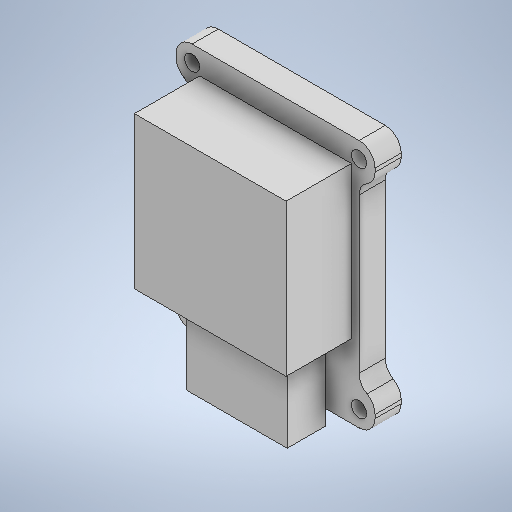
# Autodesk Inventor part: IR_cam
Saved by Autodesk Inventor 2025.3 (Build 293356000, 356)
## iProperties
Created: 2025-06-24
Part Number: IR_cam
Material: Generic
Document SubType Name: Modeling
Designer: vagrant
Density: 1 g/cm^3
Appearance: Default
Author: vagrant
Autodesk Inventor part; units mm, degrees
ref_plane "YZ Plane" through (0, 0, 0) normal (1, 0, 0) x (0, 1, 0)
ref_plane "XZ Plane" through (0, 0, 0) normal (0, 1, 0) x (-1, 0, 0)
ref_plane "XY Plane" through (0, 0, 0) normal (0, 0, 1) x (1, 0, 0)
sketch "Sketch1" plane through (0, 0, 0) normal (0, 0, 1) x (1, 0, 0)
  line L0 (-7.619, -8.598) -> (7.601, -8.598)
  line L1 (7.601, -8.598) -> (7.601, 10.452)
  line L2 (7.601, 10.452) -> (-7.619, 10.452)
  line L3 (-7.619, 10.452) -> (-7.619, -8.598)
  line L4 (-6.394, 9.217) -> (6.376, 9.217)
  line L5 (6.376, 9.217) -> (6.376, -7.363)
  line L6 (6.376, -7.363) -> (-6.394, -7.363)
  line L7 (-6.394, -7.363) -> (-6.394, 9.217)
  circle A0 centre (-6.394, 9.217) radius 0.58
  circle A1 centre (6.376, 9.217) radius 0.58
  circle A2 centre (6.376, -7.363) radius 0.58
  circle A3 centre (-6.394, -7.363) radius 0.58
  line L8 (-3.844, -9.748) -> (3.826, -9.748)
  line L9 (3.826, -9.748) -> (3.826, -8.598)
  line L10 (-3.844, -9.748) -> (-3.844, -8.598)
  line L11 (5.796, 8.637) -> (-5.814, 8.637)
  line L12 (-5.814, 8.637) -> (-5.814, -2.973)
  line L13 (-5.814, -2.973) -> (5.796, -2.973)
  line L14 (5.796, -2.973) -> (5.796, 8.637)
  line L15 (3.826, -9.748) -> (-3.844, -9.748)
  line L16 (-3.844, -9.748) -> (-3.844, -4.118)
  line L17 (-3.844, -4.118) -> (3.826, -4.118)
  line L18 (3.826, -4.118) -> (3.826, -9.748)
  line L19 (-6.394, -6.203) -> (-4.894, -6.203)
  line L20 (-4.894, -6.203) -> (-4.894, -3.703)
  line L21 (-4.894, -3.703) -> (-6.394, -3.703)
  line L22 (-6.394, -3.703) -> (-6.394, -6.203)
  line L23 (-7.619, 8.057) -> (-6.394, 8.057)
  line L24 (-6.394, 8.057) -> (-6.394, -6.783)
  line L25 (-7.619, -6.783) -> (-7.619, 8.057)
  line L26 (7.601, 8.637) -> (7.601, -6.783)
  line L27 (6.376, -6.783) -> (6.376, 8.637)
  line L28 (-6.394, 10.452) -> (-6.394, 9.797)
  line L29 (6.376, 10.452) -> (6.376, 9.797)
  line L30 (-7.619, -6.203) -> (-6.394, -6.203)
  line L31 (6.376, -6.203) -> (7.601, -6.203)
  line L32 (6.376, 8.057) -> (7.601, 8.057)
  point P0 (0, 0)
  point P1 (2.2173, 6.5337)
  point P2 (-0.009, -8.598)
  point P3 (-0.009, -9.748)
  point P4 (-6.394, -3.703)
  point P5 (-4.894, -4.953)
  point P6 (-5.644, -6.203)
  point P7 (-6.394, 8.057)
  point P8 (-7.0065, -6.783)
  point P9 (6.9885, 8.637)
  point P10 (-7.0065, -6.203)
  dimension "d16" = 1.16
  dimension "d17" = 1.16
  dimension "d0" = 15.22
  dimension "d1" = 19.05
  dimension "d14" = 12.77
  dimension "d15" = 16.58
  dimension "d18" = 1.16
  dimension "d19" = 1.16
  dimension "d23" = 1.235
  dimension "d24" = 1.225
  dimension "d47" = 1.15
  dimension "d55" = 5.63
  dimension "d60" = 1.5
  dimension "d61" = 2.5
  dimension "d64" = 2.395
  dimension "d67" = 2.395
  constraints: 66 end point, 16 point on line, 15 perpendicular, 9 parallel, 7 horizontal, 5 midpoint, 4 coincident, 2 centre point, 2 point on circle, 2 vertical alignment, 1 collinear, 4 other
  measures "d0" distance of L0.start L0.end
  measures "d1" distance of L2.end L0.start
  measures "d14" distance of L5.end L6.end
  measures "d15" distance of L4.start L6.end
  measures "d18" diameter of A2
  measures "d19" diameter of A1
  measures "d23" distance from line of L2 point (-6.394, 9.217)
  measures "d24" distance from line of L1 A1.centre
  measures "d47" distance of point (-0.009, -8.598) point (-0.009, -9.748)
  measures "d55" distance between parallel lines of L17 L15
  measures "d60" distance from line of point (-4.894, -4.953) L7
  measures "d61" distance from line of L21 point (-5.644, -6.203)
  measures "d64" distance between parallel lines of L23 L2
  measures "d67" distance from line of L0 point (-7.006, -6.203)
extrude "Extrusion1" add sketch "Sketch1" against normal blind 2 contours L3 L30 L7 A3 L6 L16 L0 | L16 L6 L18 L0 | L18 L6 A2 L5 L31 L1 L0 | L16 L17 L18 L6 | L6 A3 L7 L19 L20 L21 A0 L4 A1 L5 A2 L18 L17 L16 | L3 L23 L7 L30 | L3 L2 L28 A0 L7 L23 | L7 L21 L20 L19 | L31 L5 L32 L1 | L2 L29 A1 L4 A0 L28 | L32 L5 A1 L29 L2 L1 | L14 L13 L12 L11
extrude "Extrusion6" add sketch "Sketch1" along normal blind 5 contours L14 L13 L12 L11
extrude "Extrusion7" add sketch "Sketch1" along normal blind 2.95 contours L16 L6 L18 L0 | L0 L9 L8 L10 | L16 L17 L18 L6
extrude "Extrusion8" add sketch "Sketch1" along normal blind 1.5 contours L7 L21 L20 L19
extrude "Extrusion10" cut sketch "Sketch1" against normal blind 2 contours L3 L23 L7 L30 | L31 L5 L32 L1
fillet "Fillet13" radius 1.22 12 edges at (7.601, 10.452, -1) (7.601, 8.057, -1) (6.376, 8.057, -1) (7.601, -6.203, -1) (6.376, -6.203, -1) (7.601, -8.598, -1) (-6.394, -6.203, -1) (-7.619, -6.203, -1) (-7.619, -8.598, -1) (-7.619, 10.452, -1) (-7.619, 8.057, -1) (-6.394, 8.057, -1)
body "Solid1"
